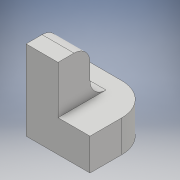
# Autodesk Inventor part: 45
Saved by Autodesk Inventor 2017 (Build 210142000, 142)
## iProperties
Part Number: 45
Material: 一般
Document SubType Name: Modeling
Designer: Brian
Density: 1 g/cm^3
Appearance: 預設
Author: Brian
Autodesk Inventor part; units mm, degrees
ref_plane "YZ Plane" through (0, 0, 0) normal (1, 0, 0) x (0, 1, 0)
ref_plane "XZ Plane" through (0, 0, 0) normal (0, 1, 0) x (-1, 0, 0)
ref_plane "XY Plane" through (0, 0, 0) normal (0, 0, 1) x (1, 0, 0)
sketch "草圖1" plane through (0, 0, 0) normal (0, 1, 0) x (-1, 0, 0)
  line L0 (0, 0) -> (-20, 0)
  line L1 (-20, 0) -> (-20, -30)
  line L2 (-20, -30) -> (0, -30)
  line L3 (0, -30) -> (0, 0)
  dimension "d0" = 30
  dimension "d1" = 20
  constraints: 8 end point, 2 parallel, 1 horizontal, 1 perpendicular
  measures "d0" distance of L0.end L1.end
  measures "d1" distance of L1.end L2.end
extrude "擠出1" add sketch "草圖1" along normal blind 20
sketch "草圖2" plane through (20, 0, -30) normal (0, 0, -1) x (-1, 0, 0)
  line L0 (20, 0) -> (0, 0) projected
  line L1 (20, 0) -> (-20, 0)
  line L2 (-20, 0) -> (-20, 40)
  line L3 (-20, 40) -> (20, 40)
  line L4 (20, 40) -> (20, 0)
  dimension "d4" = 40
  dimension "d5" = 40
  constraints: 8 end point, 2 parallel, 1 horizontal, 1 perpendicular
  measures "d4" distance of L2.end L3.end
  measures "d5" distance of L3.end L0.start
extrude "擠出2" add sketch "草圖2" along normal blind 20
fillet "圓角1" radius 10 2 edges at (10, 20, -30) (10, 20, 0)
fillet "圓角2" radius 20 1 edges at (40, 40, -40)
